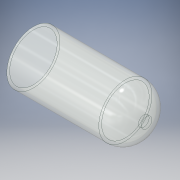
# Autodesk Inventor part: piston cup
Saved by Autodesk Inventor 2018 (Build 220112000, 112)
## iProperties
Created: 2018-03-07
Part Number: piston cup
Material: Glass
Document SubType Name: Modeling
Designer: 238438
Density: 2.18 g/cm^3
Appearance: Clear
Mass: 1.2662 g
Surface Area: 18.5276 cm^2
Volume: 0.580824 cm^3
Author: 238438
Autodesk Inventor part; units mm, degrees
ref_plane "YZ Plane" through (0, 0, 0) normal (1, 0, 0) x (0, 1, 0)
ref_plane "XZ Plane" through (0, 0, 0) normal (0, 1, 0) x (-1, 0, 0)
ref_plane "XY Plane" through (0, 0, 0) normal (0, 0, 1) x (1, 0, 0)
sketch "Sketch1" plane through (0, 0, 0) normal (1, 0, 0) x (0, 1, 0)
  circle A0 centre (0, 0) radius 5.969
  dimension "d0" = 11.938
  constraints: 1 centre point, 1 coincident
  measures "d0" diameter of A0
extrude "Extrusion1" add sketch "Sketch1" along normal blind 25.4
fillet "Fillet1" radius 4.7625 1 edges at (25.4, -5.969, 0)
shell "Shell1" thickness 0.635 removed faces 1 at (0, -1.9689, -1.3194)
body "Solid1"
